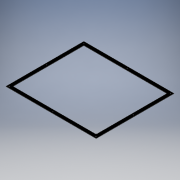
# Autodesk Inventor part: Top Cladding
Saved by Autodesk Inventor 2017.3 (Build 213256000, 256)
## iProperties
Created: 2018-10-13
Part Number: Top Cladding
Material: Aluminum 6061
Document SubType Name: Sheet Metal
Designer: Ax
Density: 2.7 g/cm^3
Sheet Metal Rule: Default_mm
Appearance: Anodized - Black
Author: Ax
Autodesk Inventor part; units mm, degrees
ref_plane "YZ Plane" through (0, 0, 0) normal (1, 0, 0) x (0, 1, 0)
ref_plane "XZ Plane" through (0, 0, 0) normal (0, 1, 0) x (-1, 0, 0)
ref_plane "XY Plane" through (0, 0, 0) normal (0, 0, 1) x (1, 0, 0)
sketch "Sketch1" plane through (0, 0, 0) normal (0, 0, 1) x (1, 0, 0)
  line L0 (-256.5, -221.5) -> (256.5, -221.5)
  line L1 (256.5, -221.5) -> (256.5, 221.5)
  line L2 (256.5, 221.5) -> (-256.5, 221.5)
  line L3 (-256.5, 221.5) -> (-256.5, -221.5)
  line L4 (-256.5, -221.5) -> (256.5, 221.5) construction
  line L5 (256.5, -221.5) -> (-256.5, 221.5) construction
  line L6 (-256.5, 211.5) -> (256.5, 211.5) construction
  line L7 (-246.5, 221.5) -> (-246.5, -221.5) construction
  line L8 (246.5, 221.5) -> (246.5, -221.5) construction
  line L9 (-256.5, -111.5) -> (256.5, -111.5) construction
  line L10 (-256.5, 141.5) -> (256.5, 141.5) construction
  circle A0 centre (-246.5, 211.5) radius 2.1
  circle A1 centre (246.5, 211.5) radius 2.1
  line L11 (-146.5, 221.5) -> (-146.5, -221.5) construction
  line L12 (0, 0) -> (0, -221.5) construction
  line L13 (146.5, 221.5) -> (146.5, -221.5) construction
  line L14 (-246.5, 70) -> (246.5, 70) construction
  line L15 (-246.5, -70) -> (246.5, -70) construction
  line L16 (-246.5, 0) -> (246.5, 0) construction
  line L17 (-246.5, -166.5) -> (246.5, -166.5) construction
  line L18 (0, 221.5) -> (0, 0) construction
  circle A2 centre (0, 211.5) radius 2.1
  line L19 (231.5, 201.5) -> (-234.5, 201.5)
  line L20 (-236.5, 199.5) -> (-236.5, -196.5)
  line L21 (-231.5, -201.5) -> (231.5, -201.5)
  line L22 (236.5, -196.5) -> (236.5, 196.5)
  arc A3 (-234.5, 201.5) -> (-236.5, 199.5) centre (-234.5, 199.5) ccw
  arc A4 (236.5, 196.5) -> (231.5, 201.5) centre (231.5, 196.5) ccw
  arc A5 (231.5, -201.5) -> (236.5, -196.5) centre (231.5, -196.5) ccw
  arc A6 (-236.5, -196.5) -> (-231.5, -201.5) centre (-231.5, -196.5) ccw
  circle A7 centre (246.5, 0) radius 2.1
  circle A8 centre (246.5, -212.8645) radius 2.1
  circle A9 centre (-246.5, -212.8645) radius 2.1
  circle A10 centre (0, -211.5) radius 2.1
  circle A11 centre (-246.5, 0) radius 2.1
  dimension "d0" = 513
  dimension "d1" = 443
  dimension "d2" = 10
  dimension "d3" = 10
  dimension "d4" = 10
  dimension "d5" = 110
  dimension "d6" = 80
  dimension "d7" = 110
  dimension "d8" = 110
  dimension "d9" = 70
  dimension "d10" = 55
  dimension "d23" = 10
  dimension "d24" = 10
  dimension "d25" = 20
  dimension "d26" = 10
  dimension "d27" = 2
  dimension "d28" = 5
  dimension "d29" = 4.2
  dimension "d30" = 10
  measures "d0" distance of L1.end L2.end
  measures "d1" distance of L0.end L1.end
  measures "d2" distance of L2.end L6.start
  measures "d3" distance of L0.start L7.end
  measures "d4" distance of L0.end L8.end
  measures "d5" distance of L0.end L9.end
  measures "d6" distance of L10.end L1.end
  measures "d7" distance of L0.start L11.end
  measures "d8" distance of L13.end L0.end
  measures "d9" vertical distance of L12.start L14.start
  measures "d10" vertical distance of L0.end L17.end
  measures "d23" distance between parallel lines of L6 L19
  measures "d24" distance between parallel lines of L8 L22
  measures "d25" distance between parallel lines of L0 L21
  measures "d26" distance between parallel lines of L20 L7
  measures "d27" radius of A3
  measures "d28" radius of A4
  measures "d29" diameter of A2
  measures "d30" distance from line of L0 A10.centre
extrude "Plate6" add sketch "Sketch1" along normal blind 1.5
equation "\"BendRadius\" = Thickness"
equation "\"BendReliefWidth\" = Thickness"
equation "\"BendReliefDepth\" = 0.5 * Thickness"
equation "\"CornerReliefSize\" = 4 * Thickness"
equation "\"MinimumRemnant\" = 2 * Thickness"
equation "\"TransitionRadius\" = BendRadius"
equation "\"JacobiRadiusSize\" = BendRadius"
equation "\"GapSize\" = Thickness"
equation "\"d12\" = BendRadius"
equation "\"d13\" = BendRadius"
equation "\"d16\" = BendRadius"
equation "\"d19\" = BendRadius"
equation "\"d20\" = BendRadius"
equation "\"d31\" = BendRadius"
equation "\"Thickness\" = 1.5"
body "Solid6"
